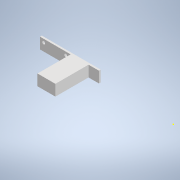
# Autodesk Inventor part: sujetador_motor
Saved by Autodesk Inventor 2022 (Build 260153000, 153)
## iProperties
Created: 2022-03-16
Part Number: sujetador_motor
Material: Generic
Document SubType Name: Modeling
Designer: katha
Density: 1 g/cm^3
Appearance: Default
Author: katha
Autodesk Inventor part; units mm, degrees
ref_plane "YZ Plane" through (0, 0, 0) normal (1, 0, 0) x (0, 1, 0)
ref_plane "XZ Plane" through (0, 0, 0) normal (0, 1, 0) x (-1, 0, 0)
ref_plane "XY Plane" through (0, 0, 0) normal (0, 0, 1) x (1, 0, 0)
sketch "Sketch1" plane through (0, 0, 0) normal (0, 0, 1) x (1, 0, 0)
  circle A0 centre (-173.3589, -112.9) radius 2 projected
  circle A1 centre (-143.3589, -112.9) radius 2 projected
  circle A2 centre (-173.3589, -112.9) radius 2
  circle A3 centre (-143.3589, -112.9) radius 2
  line L0 (-178.3589, -108.4) -> (-98.3589, -108.4)
  line L1 (-98.3589, -108.4) -> (-98.3589, -123.4)
  line L2 (-98.3589, -123.4) -> (-178.3589, -123.4)
  line L3 (-178.3589, -123.4) -> (-178.3589, -108.4)
  point P0 (0, 0)
  dimension "d0" = 4
  dimension "d1" = 4
  dimension "d2" = 15
  dimension "d3" = 80
  dimension "d4" = 4.5
  dimension "d5" = 5
  constraints: 8 end point, 2 centre point, 2 coincident, 2 parallel, 1 horizontal, 1 perpendicular
  measures "d0" diameter of A2
  measures "d1" diameter of A3
  measures "d2" distance between parallel lines of L2 L0
  measures "d3" distance between parallel lines of L1 L3
  measures "d4" distance from line of L0 A0.centre
  measures "d5" distance from line of L3 A0.centre
extrude "Extrusion1" add sketch "Sketch1" along normal blind 2.5
sketch "Sketch2" plane through (0, 0, 2.5) normal (0, 0, 1) x (1, 0, 0)
  line L0 (-178.3589, -123.4) -> (-98.3589, -123.4) projected
  line L1 (-98.3589, -123.4) -> (-98.3589, -108.4) projected
  line L2 (-98.3589, -108.4) -> (-178.3589, -108.4) projected
  line L3 (-178.3589, -108.4) -> (-178.3589, -123.4) projected
  circle A0 centre (-143.3589, -112.9) radius 2 projected
  circle A1 centre (-173.3589, -112.9) radius 2 projected
  line L4 (-122.2642, -87.4) -> (-126.8642, -87.4) projected
  line L5 (-124.5642, -87.4) -> (-124.5642, -147.4431) construction
  line L6 (-124.5642, -115.9) -> (-114.5642, -115.9) construction
  line L7 (-98.3589, -108.4) -> (-178.3589, -108.4) projected
  line L8 (-114.5642, -115.9) -> (-114.5642, -123.4)
  line L9 (-114.5642, -115.9) -> (-114.5642, -108.4)
  line L10 (-134.5642, -115.9) -> (-134.5642, -123.4)
  line L11 (-134.5642, -115.9) -> (-134.5642, -108.4)
  line L12 (-114.5642, -123.4) -> (-134.5642, -123.4)
  line L13 (-178.3589, -123.4) -> (-98.3589, -123.4) projected
  line L14 (-114.5642, -108.4) -> (-134.5642, -108.4)
  point P0 (0, 0)
  point P1 (-112.4142, -124.5353)
  point P2 (-112.4142, -107.2647)
  dimension "d8" = 10
  constraints: 16 end point, 4 symmetric about line, 3 point on line, 2 collinear, 2 vertical, 1 horizontal, 1 midpoint
  measures "d8" distance of L6.start L6.end
extrude "Extrusion2" add sketch "Sketch2" along normal blind 45 contours L10 L11 L2 L9 L8 L0
sketch "Sketch3" plane through (-178.3589, -123.4, 0) normal (0, -1, 0) x (1, 0, 0)
  circle A0 centre (53.7947, 57.0153) radius 2.3 construction
  line L0 (53.7947, 57.0153) -> (53.7947, 47.7653) construction
  line L1 (53.7947, 57.0153) -> (65.8947, 57.0153) construction
  line L2 (53.7947, 47.7653) -> (61.5952, 47.7653) construction
  line L3 (53.7947, 47.7653) -> (45.9942, 47.7653) construction
  line L4 (53.7947, 66.2653) -> (61.5952, 66.2653) construction
  line L5 (53.7947, 66.2653) -> (45.9942, 66.2653) construction
  arc A1 (45.9942, 66.2653) -> (45.9942, 47.7653) centre (53.7947, 57.0153) ccw construction
  arc A2 (61.5952, 47.7653) -> (61.5952, 66.2653) centre (53.7947, 57.0153) ccw construction
  line L6 (61.6679, 66.4653) -> (53.9215, 66.4653)
  line L7 (53.9215, 66.4653) -> (45.9215, 66.4653)
  arc A3 (45.9215, 66.4653) -> (45.9215, 47.5653) centre (53.7947, 57.0153) ccw
  line L8 (45.9215, 47.5653) -> (53.7947, 47.5653)
  line L9 (53.7947, 47.5653) -> (61.6679, 47.5653)
  arc A4 (61.6679, 47.5653) -> (61.6679, 66.4653) centre (53.7947, 57.0153) ccw
  line L10 (62.1934, 67.9653) -> (59.2947, 67.9653)
  arc A5 (45.396, 67.9653) -> (45.396, 46.0653) centre (53.7947, 57.0153) ccw
  line L11 (45.396, 46.0653) -> (53.7947, 46.0653)
  line L12 (53.7947, 46.0653) -> (62.1934, 46.0653)
  arc A6 (62.1934, 46.0653) -> (62.1934, 67.9653) centre (53.7947, 57.0153) ccw
  line L13 (57.7947, 66.4653) -> (57.7947, 74.4653)
  line L14 (49.7947, 66.4653) -> (49.7947, 74.4653)
  line L15 (59.2947, 67.9653) -> (59.2947, 74.4653)
  line L16 (48.2947, 67.9653) -> (48.2947, 74.4653)
  line L17 (48.2947, 74.4653) -> (49.7947, 74.4653)
  line L18 (57.7947, 74.4653) -> (59.2947, 74.4653)
  line L19 (48.2947, 67.9653) -> (45.396, 67.9653)
  point P0 (178.3589, 0)
  dimension "d11" = 9.25
  dimension "d12" = 12.1
  dimension "d13" = 0.2
  dimension "d14" = 1.5
  dimension "d15" = 8
  dimension "d16" = 4
  dimension "d17" = 1.5
  dimension "d18" = 1.5
  constraints: 40 end point, 13 point on circle, 6 centre point, 6 symmetric about line, 3 horizontal, 2 parallel, 2 vertical, 1 coincident, 1 collinear, 1 midpoint, 8 other
  measures "d11" distance of L0.start L0.end
  measures "d12" distance of L0.start L1.end
  measures "d13" radial gap between concentric circles of A2 A4
  measures "d14" radial gap between concentric circles of A4 A6
  measures "d15" distance of L13.start L13.end
  measures "d16" distance between parallel lines of L13 L0
  measures "d17" distance between parallel lines of L13 L15
  measures "d18" distance between parallel lines of L14 L16
extrude "Extrusion3" add sketch "Sketch3" against normal blind 15 contours L6 L13 L18 L15 L10 A6 L12 L11 A5 L19 L16 L17 L14 L7 A3 L8 L9 A4
body "Solid1"
